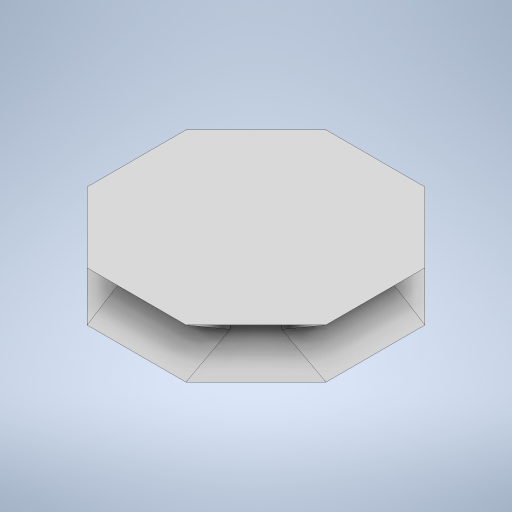
# Autodesk Inventor part: 팔각형 OV-PAM 층 한개
Saved by Autodesk Inventor 2024 (Build 280153000, 153)
## iProperties
Created: 2023-06-16
Part Number: 팔각형 OV-PAM 층 한개
Material: 일반
Document SubType Name: Modeling
Designer: jsw
Density: 1 g/cm^3
Appearance: 기본값
Mass: 35.2679 g
Surface Area: 129.281 cm^2
Volume: 35.2679 cm^3
Author: jsw
Autodesk Inventor part; units mm, degrees
ref_plane "YZ Plane" through (0, 0, 0) normal (1, 0, 0) x (0, 1, 0)
ref_plane "XZ Plane" through (0, 0, 0) normal (0, 1, 0) x (-1, 0, 0)
ref_plane "XY Plane" through (0, 0, 0) normal (0, 0, 1) x (1, 0, 0)
sketch "스케치1" plane through (0, 0, 0) normal (0, 1, 0) x (-1, 0, 0)
  line L0 (-32.5919, 13.5) -> (-13.5, 32.5919)
  line L1 (-13.5, 32.5919) -> (13.5, 32.5919)
  line L2 (13.5, 32.5919) -> (32.5919, 13.5)
  line L3 (32.5919, 13.5) -> (32.5919, -13.5)
  line L4 (32.5919, -13.5) -> (13.5, -32.5919)
  line L5 (13.5, -32.5919) -> (-13.5, -32.5919)
  line L6 (-13.5, -32.5919) -> (-32.5919, -13.5)
  line L7 (-32.5919, -13.5) -> (-32.5919, 13.5)
  line L8 (-13.8314, 33.3919) -> (13.8314, 33.3919)
  line L9 (13.8314, 33.3919) -> (33.3919, 13.8314)
  line L10 (33.3919, 13.8314) -> (33.3919, -13.8314)
  line L11 (33.3919, -13.8314) -> (13.8314, -33.3919)
  line L12 (13.8314, -33.3919) -> (-13.8314, -33.3919)
  line L13 (-13.8314, -33.3919) -> (-33.3919, -13.8314)
  line L14 (-33.3919, -13.8314) -> (-33.3919, 13.8314)
  line L15 (-33.3919, 13.8314) -> (-13.8314, 33.3919)
  point P0 (0, 0)
  point P1 (0, 0)
  point P2 (0, 0)
  dimension "d0" = 27
  dimension "d2" = 0.8
  constraints: 32 end point, 2 coincident, 2 horizontal, 34 other
  measures "d0" distance of L0.end L1.end
  measures "d2" distance between parallel lines of L10 L3
extrude "돌출2" add sketch "스케치1" along normal blind 6.93 contours L0 L1 L2 L3 L4 L5 L6 L7 | L8 L9 L10 L11 L12 L13 L14 L15
ref_plane "작업 평면2" through (33.3919, 0, 13.8314) normal (-0.5, -0.8660254, 0) x (0, 0, -1)
sketch "스케치3" plane through (33.3919, 0, 13.8314) normal (1, 0, 0) x (0, 0, -1)
  line L0 (0, 0) -> (0, 6.93) projected
  line L1 (0, 6.93) -> (27.6627, 6.93) projected
  line L2 (0, 0) -> (27.6627, 0)
  line L3 (27.6627, 0) -> (27.6627, 6.93)
  line L4 (27.6627, 6.93) -> (0, 6.93)
  line L5 (0, 6.93) -> (0, 0)
  line L6 (0, 6.93) -> (-11.0903, 6.93)
  line L7 (-19.5605, 6.93) -> (0, 6.93) projected
  line L8 (0, 0) -> (-11.0903, 6.93)
  line L9 (27.6627, 6.93) -> (38.7531, 6.93)
  line L10 (38.7531, 6.93) -> (27.6627, 0)
  point P0 (13.8314, 0)
  dimension "d18" = 148
  dimension "d43" = 148
  constraints: 16 end point, 2 parallel, 2 point on line, 1 horizontal, 1 perpendicular
  measures "d18" angle of L2 L10
  measures "d43" angle of L8 L2
extrude "돌출4" cut sketch "스케치3" against normal up to surface surface through (33.3919, 0, 13.8314) normal (-0.5, -0.8660254, 0)
sketch "스케치4" plane through (13.8314, 0, 33.3919) normal (0.7071068, 0, 0.7071068) x (0.7071068, 0, -0.7071068)
  line L0 (0, 0) -> (0, 6.93) projected
  line L1 (27.6627, 0) -> (27.6627, 6.93) projected
  line L2 (0, 0) -> (27.6627, 0)
  line L3 (27.6627, 0) -> (27.6627, 6.93)
  line L4 (27.6627, 6.93) -> (0, 6.93)
  line L5 (0, 6.93) -> (0, 0)
  line L6 (27.6627, 0) -> (18.9404, 6.93)
  line L7 (27.6627, 0) -> (0, 0) projected
  line L8 (0, 0) -> (8.7224, 6.93)
  line L9 (27.6627, 6.93) -> (0, 6.93) projected
  line L10 (8.7224, 6.93) -> (0, 6.93)
  line L11 (18.9404, 6.93) -> (27.6627, 6.93)
  line L12 (13.8314, 0) -> (13.8314, 6.93)
  point P0 (8.7224, 6.93)
  point P1 (27.6627, 0)
  point P2 (13.8314, 6.93)
  dimension "d41" = 10.218
  dimension "d42" = 5.109
  constraints: 18 end point, 3 point on line, 2 midpoint, 2 parallel, 2 perpendicular, 1 collinear, 1 horizontal
  measures "d41" distance of L8.end L6.end
  measures "d42" distance of point (13.831, 6.93) L6.end
ref_plane "작업 평면3" through (13.8314, 0, 33.3919) normal (0.3535534, 0.8660254, 0.3535534) x (0.7071068, 0, -0.7071068)
extrude "돌출5" cut sketch "스케치4" against normal up to surface contours L8 L4 L12 L2 | L12 L4 L6 L2 surface through (13.8314, 0, 33.3919) normal (0.3535534, 0.8660254, 0.3535534)
pattern_circular "원형 패턴1" count 4 over 360 about axis through (0, -10, 0) along (0, 1, 0) of "돌출4"
pattern_circular "원형 패턴2" count 4 over 360 about axis through (0, -10, 0) along (0, 1, 0) of "돌출5"
mirror "미러5" about plane through (0, 6.93, 0) normal (0, 1, 0) of "돌출2", "돌출5", "원형 패턴2", "돌출4", "원형 패턴1"
ref_plane "작업 평면5" through (-13.8314, 6.93, -33.3919) normal (0, 1, 0) x (1, 0, 0)
equation "\"d42\" = 0.5 * d41"
